Autodesk Fusion 360 part; units mm, degrees
(part 5 of 18)
  arc A132 (38.8971, -63.5184) -> (40.0971, -63.5184) centre (39.4971, -63.5184) ccw
  arc A133 (40.0971, -63.5184) -> (38.8971, -63.5184) centre (39.4971, -63.5184) ccw
  arc A134 (43.5971, -80.3272) -> (42.3971, -80.3272) centre (42.9971, -80.3272) ccw
  arc A135 (42.3971, -80.3272) -> (43.5971, -80.3272) centre (42.9971, -80.3272) ccw
  arc A136 (38.8971, -82.5812) -> (40.0971, -82.5812) centre (39.4971, -82.5812) ccw
  arc A137 (40.0971, -82.5812) -> (38.8971, -82.5812) centre (39.4971, -82.5812) ccw
  arc A138 (24.547, -80.3272) -> (23.347, -80.3272) centre (23.947, -80.3272) ccw
  arc A139 (23.347, -80.3272) -> (24.547, -80.3272) centre (23.947, -80.3272) ccw
  arc A140 (21.047, -82.5812) -> (19.847, -82.5812) centre (20.447, -82.5812) ccw
  arc A141 (19.847, -82.5812) -> (21.047, -82.5812) centre (20.447, -82.5812) ccw
  arc A142 (5.497, -80.3272) -> (4.297, -80.3272) centre (4.897, -80.3272) ccw
  arc A143 (4.297, -80.3272) -> (5.497, -80.3272) centre (4.897, -80.3272) ccw
  arc A144 (0.797, -82.5812) -> (1.997, -82.5812) centre (1.397, -82.5812) ccw
  arc A145 (1.997, -82.5812) -> (0.797, -82.5812) centre (1.397, -82.5812) ccw
  arc A146 (62.6471, -23.1516) -> (61.4471, -23.1516) centre (62.0471, -23.1516) ccw
  arc A147 (61.4471, -23.1516) -> (62.6471, -23.1516) centre (62.0471, -23.1516) ccw
  arc A148 (57.9471, -25.4057) -> (59.1471, -25.4057) centre (58.5471, -25.4057) ccw
  arc A149 (59.1471, -25.4057) -> (57.9471, -25.4057) centre (58.5471, -25.4057) ccw
  arc A150 (42.3971, -42.2017) -> (43.5971, -42.2017) centre (42.9971, -42.2017) ccw
  arc A151 (43.5971, -42.2017) -> (42.3971, -42.2017) centre (42.9971, -42.2017) ccw
  arc A152 (38.8971, -44.4557) -> (40.0971, -44.4557) centre (39.4971, -44.4557) ccw
  arc A153 (40.0971, -44.4557) -> (38.8971, -44.4557) centre (39.4971, -44.4557) ccw
  arc A154 (43.5971, -23.1516) -> (42.3971, -23.1516) centre (42.9971, -23.1516) ccw
  arc A155 (42.3971, -23.1516) -> (43.5971, -23.1516) centre (42.9971, -23.1516) ccw
  arc A156 (40.0971, -25.4057) -> (38.8971, -25.4057) centre (39.4971, -25.4057) ccw
  arc A157 (38.8971, -25.4057) -> (40.0971, -25.4057) centre (39.4971, -25.4057) ccw
  arc A158 (24.547, -23.1516) -> (23.347, -23.1516) centre (23.947, -23.1516) ccw
  arc A159 (23.347, -23.1516) -> (24.547, -23.1516) centre (23.947, -23.1516) ccw
  arc A160 (21.047, -25.4057) -> (19.847, -25.4057) centre (20.447, -25.4057) ccw
  arc A161 (19.847, -25.4057) -> (21.047, -25.4057) centre (20.447, -25.4057) ccw
  arc A162 (24.547, -61.2644) -> (23.347, -61.2644) centre (23.947, -61.2644) ccw
  arc A163 (23.347, -61.2644) -> (24.547, -61.2644) centre (23.947, -61.2644) ccw
  arc A164 (19.847, -63.5184) -> (21.047, -63.5184) centre (20.447, -63.5184) ccw
  arc A165 (21.047, -63.5184) -> (19.847, -63.5184) centre (20.447, -63.5184) ccw
  arc A166 (24.547, -42.2017) -> (23.347, -42.2017) centre (23.947, -42.2017) ccw
  arc A167 (23.347, -42.2017) -> (24.547, -42.2017) centre (23.947, -42.2017) ccw
  arc A168 (19.847, -44.4557) -> (21.047, -44.4557) centre (20.447, -44.4557) ccw
  arc A169 (21.047, -44.4557) -> (19.847, -44.4557) centre (20.447, -44.4557) ccw
  arc A170 (4.297, -23.1516) -> (5.497, -23.1516) centre (4.897, -23.1516) ccw
  arc A171 (5.497, -23.1516) -> (4.297, -23.1516) centre (4.897, -23.1516) ccw
  arc A172 (0.797, -25.4057) -> (1.997, -25.4057) centre (1.397, -25.4057) ccw
  arc A173 (1.997, -25.4057) -> (0.797, -25.4057) centre (1.397, -25.4057) ccw
  arc A174 (5.497, -42.2017) -> (4.297, -42.2017) centre (4.897, -42.2017) ccw
  arc A175 (4.297, -42.2017) -> (5.497, -42.2017) centre (4.897, -42.2017) ccw
  arc A176 (0.797, -44.4557) -> (1.997, -44.4557) centre (1.397, -44.4557) ccw
  arc A177 (1.997, -44.4557) -> (0.797, -44.4557) centre (1.397, -44.4557) ccw
  arc A178 (5.497, -61.2644) -> (4.297, -61.2644) centre (4.897, -61.2644) ccw
  arc A179 (4.297, -61.2644) -> (5.497, -61.2644) centre (4.897, -61.2644) ccw
  arc A180 (0.797, -63.5184) -> (1.997, -63.5184) centre (1.397, -63.5184) ccw
  arc A181 (1.997, -63.5184) -> (0.797, -63.5184) centre (1.397, -63.5184) ccw
  arc A182 (215.0474, -61.2644) -> (213.8474, -61.2644) centre (214.4474, -61.2644) ccw
  arc A183 (213.8474, -61.2644) -> (215.0474, -61.2644) centre (214.4474, -61.2644) ccw
  arc A184 (210.3474, -63.5184) -> (211.5474, -63.5184) centre (210.9474, -63.5184) ccw
  arc A185 (211.5474, -63.5184) -> (210.3474, -63.5184) centre (210.9474, -63.5184) ccw
  arc A186 (213.8474, -42.2017) -> (215.0474, -42.2017) centre (214.4474, -42.2017) ccw
  arc A187 (215.0474, -42.2017) -> (213.8474, -42.2017) centre (214.4474, -42.2017) ccw
  arc A188 (210.3474, -44.4557) -> (211.5474, -44.4557) centre (210.9474, -44.4557) ccw
  arc A189 (211.5474, -44.4557) -> (210.3474, -44.4557) centre (210.9474, -44.4557) ccw
  arc A190 (213.8474, -23.1516) -> (215.0474, -23.1516) centre (214.4474, -23.1516) ccw
  arc A191 (215.0474, -23.1516) -> (213.8474, -23.1516) centre (214.4474, -23.1516) ccw
  arc A192 (211.5474, -25.4057) -> (210.3474, -25.4057) centre (210.9474, -25.4057) ccw
  arc A193 (210.3474, -25.4057) -> (211.5474, -25.4057) centre (210.9474, -25.4057) ccw
  arc A194 (215.0474, -80.3272) -> (213.8474, -80.3272) centre (214.4474, -80.3272) ccw
  arc A195 (213.8474, -80.3272) -> (215.0474, -80.3272) centre (214.4474, -80.3272) ccw
  arc A196 (210.3474, -82.5812) -> (211.5474, -82.5812) centre (210.9474, -82.5812) ccw
  arc A197 (211.5474, -82.5812) -> (210.3474, -82.5812) centre (210.9474, -82.5812) ccw
  arc A198 (194.7974, -42.2017) -> (195.9974, -42.2017) centre (195.3974, -42.2017) ccw
  arc A199 (195.9974, -42.2017) -> (194.7974, -42.2017) centre (195.3974, -42.2017) ccw
  arc A200 (191.2974, -44.4557) -> (192.4974, -44.4557) centre (191.8974, -44.4557) ccw
  arc A201 (192.4974, -44.4557) -> (191.2974, -44.4557) centre (191.8974, -44.4557) ccw
  arc A202 (176.9224, -4.318) -> (175.1224, -4.318) centre (176.0224, -4.318) ccw
  arc A203 (175.1224, -4.318) -> (176.9224, -4.318) centre (176.0224, -4.318) ccw
  line L3366 (172.5823, -5.218) -> (172.5823, -3.418)
  line L3367 (174.3823, -3.418) -> (174.3823, -5.218)
  line L3368 (172.5823, -3.418) -> (174.3823, -3.418)
  line L3369 (174.3823, -5.218) -> (172.5823, -5.218)
  line L3370 (190.2943, -3.2705) -> (190.5139, -3.4901)
  line L3371 (190.2943, -5.4097) -> (189.9943, -5.4901)
  line L3372 (190.5943, -3.7901) -> (190.5943, -4.8901)
  line L3373 (189.4747, -3.4901) -> (189.6943, -3.2705)
  line L3374 (189.9943, -5.4901) -> (189.6943, -5.4097)
  line L3375 (189.3943, -3.7901) -> (189.4747, -3.4901)
  line L3376 (190.5139, -3.4901) -> (190.5943, -3.7901)
  line L3377 (189.6943, -5.4097) -> (189.4747, -5.1901)
  line L3378 (189.6943, -3.2705) -> (189.9943, -3.1901)
  line L3379 (189.9943, -3.1901) -> (190.2943, -3.2705)
  line L3380 (189.4747, -5.1901) -> (189.3943, -4.8901)
  line L3381 (189.3943, -4.8901) -> (189.3943, -3.7901)
  line L3382 (190.5139, -5.1901) -> (190.2943, -5.4097)
  line L3383 (190.5943, -4.8901) -> (190.5139, -5.1901)
  line L3384 (180.7544, -4.8901) -> (180.7544, -3.7901)
  line L3385 (181.0545, -3.2705) -> (181.3545, -3.1901)
  line L3386 (181.6545, -3.2705) -> (181.8741, -3.4901)
  line L3387 (181.8741, -5.1901) -> (181.6545, -5.4097)
  line L3388 (181.3545, -5.4901) -> (181.0545, -5.4097)
  line L3389 (180.8348, -5.1901) -> (180.7544, -4.8901)
  line L3390 (180.7544, -3.7901) -> (180.8348, -3.4901)
  line L3391 (181.3545, -3.1901) -> (181.6545, -3.2705)
  line L3392 (181.6545, -5.4097) -> (181.3545, -5.4901)
  line L3393 (181.8741, -3.4901) -> (181.9545, -3.7901)
  line L3394 (180.8348, -3.4901) -> (181.0545, -3.2705)
  line L3395 (181.0545, -5.4097) -> (180.8348, -5.1901)
  line L3396 (181.9545, -3.7901) -> (181.9545, -4.8901)
  line L3397 (181.9545, -4.8901) -> (181.8741, -5.1901)
  line L3398 (189.6943, -1.1096) -> (189.4747, -0.89)
  line L3399 (189.4747, 0.51) -> (189.6943, 0.7297)
  line L3400 (190.2943, 0.7297) -> (190.5139, 0.51)
  line L3401 (189.3943, -0.59) -> (189.3943, 0.21)
  line L3402 (189.4747, -0.89) -> (189.3943, -0.59)
  line L3403 (190.5943, -0.59) -> (190.5139, -0.89)
  line L3404 (190.2943, -1.1096) -> (189.9943, -1.19)
  line L3405 (189.3943, 0.21) -> (189.4747, 0.51)
  line L3406 (189.6943, 0.7297) -> (189.9943, 0.81)
  line L3407 (190.5139, 0.51) -> (190.5943, 0.21)
  line L3408 (189.9943, -1.19) -> (189.6943, -1.1096)
  line L3409 (190.5139, -0.89) -> (190.2943, -1.1096)
  line L3410 (190.5943, 0.21) -> (190.5943, -0.59)
  line L3411 (189.9943, 0.81) -> (190.2943, 0.7297)
  line L3412 (180.8348, -0.89) -> (180.7544, -0.59)
  line L3413 (181.0545, 0.7297) -> (181.3545, 0.81)
  line L3414 (181.9545, -0.59) -> (181.8741, -0.89)
  line L3415 (181.6545, -1.1096) -> (181.3545, -1.19)
  line L3416 (181.3545, -1.19) -> (181.0545, -1.1096)
  line L3417 (181.0545, -1.1096) -> (180.8348, -0.89)
  line L3418 (181.6545, 0.7297) -> (181.8741, 0.51)
  line L3419 (180.7544, 0.21) -> (180.8348, 0.51)
  line L3420 (181.8741, 0.51) -> (181.9545, 0.21)
  line L3421 (181.9545, 0.21) -> (181.9545, -0.59)
  line L3422 (180.8348, 0.51) -> (181.0545, 0.7297)
  line L3423 (181.8741, -0.89) -> (181.6545, -1.1096)
  line L3424 (181.3545, 0.81) -> (181.6545, 0.7297)
  line L3425 (180.7544, -0.59) -> (180.7544, 0.21)
  arc A204 (10.6139, -8.0011) -> (8.7123, -8.0011) centre (9.6631, -8.0011) ccw
  arc A205 (8.7123, -8.0011) -> (10.6139, -8.0011) centre (9.6631, -8.0011) ccw
  line L3426 (10.6139, -8.0011) -> (10.6139, -8.0011)
  line L3427 (10.6139, -5.4611) -> (10.6139, -5.4611)
  arc A206 (10.6139, -5.4611) -> (8.7123, -5.4611) centre (9.6631, -5.4611) ccw
  arc A207 (8.7123, -5.4611) -> (10.6139, -5.4611) centre (9.6631, -5.4611) ccw
  arc A208 (10.6139, -2.9211) -> (8.7123, -2.9211) centre (9.6631, -2.9211) ccw
  arc A209 (8.7123, -2.9211) -> (10.6139, -2.9211) centre (9.6631, -2.9211) ccw
  line L3428 (10.6139, -2.9211) -> (10.6139, -2.9211)
  arc A210 (-5.7879, -8.0011) -> (-3.8863, -8.0011) centre (-4.8371, -8.0011) ccw
  arc A211 (-3.8863, -8.0011) -> (-5.7879, -8.0011) centre (-4.8371, -8.0011) ccw
  arc A212 (-3.8863, -2.9211) -> (-5.7879, -2.9211) centre (-4.8371, -2.9211) ccw
  arc A213 (-5.7879, -2.9211) -> (-3.8863, -2.9211) centre (-4.8371, -2.9211) ccw
  line L3429 (4.2137, 0.039) -> (4.1223, -0.4205)
  line L3430 (4.1223, 0.4985) -> (4.2137, 0.039)
  line L3431 (3.4725, 1.1484) -> (3.862, 0.8881)
  line L3432 (0.4638, 0.8881) -> (0.8534, 1.1484)
  line L3433 (3.0129, -1.1618) -> (1.3129, -1.1618)
  line L3434 (0.8534, 1.1484) -> (1.3129, 1.2398)
  line L3435 (3.4725, -1.0704) -> (3.0129, -1.1618)
  line L3436 (0.4638, -0.8101) -> (0.2035, -0.4205)
  line L3437 (3.862, 0.8881) -> (4.1223, 0.4985)
  line L3438 (0.1121, 0.039) -> (0.2035, 0.4985)
  line L3439 (0.2035, 0.4985) -> (0.4638, 0.8881)
  line L3440 (0.8534, -1.0704) -> (0.4638, -0.8101)
  line L3441 (1.3129, 1.2398) -> (3.0129, 1.2398)
  line L3442 (4.1223, -0.4205) -> (3.862, -0.8101)
  line L3443 (1.3129, -1.1618) -> (0.8534, -1.0704)
  line L3444 (3.862, -0.8101) -> (3.4725, -1.0704)
  line L3445 (3.0129, 1.2398) -> (3.4725, 1.1484)
  line L3446 (0.2035, -0.4205) -> (0.1121, 0.039)
  line L3447 (3.4725, -9.8516) -> (3.862, -10.1119)
  line L3448 (0.1121, -10.961) -> (0.2035, -10.5015)
  line L3449 (0.8534, -9.8516) -> (1.3129, -9.7602)
  line L3450 (1.3129, -12.1618) -> (0.8534, -12.0704)
  line L3451 (0.4638, -10.1119) -> (0.8534, -9.8516)
  line L3452 (1.3129, -9.7602) -> (3.0129, -9.7602)
  line L3453 (0.8534, -12.0704) -> (0.4638, -11.8101)
  line L3454 (3.4725, -12.0704) -> (3.0129, -12.1618)
  line L3455 (3.0129, -9.7602) -> (3.4725, -9.8516)
  line L3456 (4.1223, -11.4205) -> (3.862, -11.8101)
  line L3457 (4.2137, -10.961) -> (4.1223, -11.4205)
  line L3458 (0.4638, -11.8101) -> (0.2035, -11.4205)
  line L3459 (3.0129, -12.1618) -> (1.3129, -12.1618)
  line L3460 (0.2035, -11.4205) -> (0.1121, -10.961)
  line L3461 (3.862, -10.1119) -> (4.1223, -10.5015)
  line L3462 (0.2035, -10.5015) -> (0.4638, -10.1119)
  line L3463 (4.1223, -10.5015) -> (4.2137, -10.961)
  line L3464 (3.862, -11.8101) -> (3.4725, -12.0704)
  arc A214 (196.0482, -61.2644) -> (194.7466, -61.2644) centre (195.3974, -61.2644) ccw
  arc A215 (194.7466, -61.2644) -> (196.0482, -61.2644) centre (195.3974, -61.2644) ccw
  arc A216 (191.2466, -63.5184) -> (192.5482, -63.5184) centre (191.8974, -63.5184) ccw
  arc A217 (192.5482, -63.5184) -> (191.2466, -63.5184) centre (191.8974, -63.5184) ccw
  arc A218 (175.6966, -80.3272) -> (176.9982, -80.3272) centre (176.3474, -80.3272) ccw
  arc A219 (176.9982, -80.3272) -> (175.6966, -80.3272) centre (176.3474, -80.3272) ccw
  arc A220 (172.1965, -82.5812) -> (173.4981, -82.5812) centre (172.8473, -82.5812) ccw
  arc A221 (173.4981, -82.5812) -> (172.1965, -82.5812) centre (172.8473, -82.5812) ccw
  arc A222 (175.6966, -61.2644) -> (176.9982, -61.2644) centre (176.3474, -61.2644) ccw
  arc A223 (176.9982, -61.2644) -> (175.6966, -61.2644) centre (176.3474, -61.2644) ccw
  arc A224 (173.4981, -63.5184) -> (172.1965, -63.5184) centre (172.8473, -63.5184) ccw
  arc A225 (172.1965, -63.5184) -> (173.4981, -63.5184) centre (172.8473, -63.5184) ccw
  arc A226 (176.9982, -42.2017) -> (175.6966, -42.2017) centre (176.3474, -42.2017) ccw
  arc A227 (175.6966, -42.2017) -> (176.9982, -42.2017) centre (176.3474, -42.2017) ccw
  arc A228 (172.1965, -44.4557) -> (173.4981, -44.4557) centre (172.8473, -44.4557) ccw
  arc A229 (173.4981, -44.4557) -> (172.1965, -44.4557) centre (172.8473, -44.4557) ccw
  arc A230 (176.9982, -23.1516) -> (175.6966, -23.1516) centre (176.3474, -23.1516) ccw
  arc A231 (175.6966, -23.1516) -> (176.9982, -23.1516) centre (176.3474, -23.1516) ccw
  arc A232 (172.1965, -25.4057) -> (173.4981, -25.4057) centre (172.8473, -25.4057) ccw
  arc A233 (173.4981, -25.4057) -> (172.1965, -25.4057) centre (172.8473, -25.4057) ccw
  arc A234 (157.9481, -80.3272) -> (156.6465, -80.3272) centre (157.2973, -80.3272) ccw
  arc A235 (156.6465, -80.3272) -> (157.9481, -80.3272) centre (157.2973, -80.3272) ccw
  arc A236 (153.1465, -82.5812) -> (154.4481, -82.5812) centre (153.7973, -82.5812) ccw
  arc A237 (154.4481, -82.5812) -> (153.1465, -82.5812) centre (153.7973, -82.5812) ccw
  arc A238 (157.9481, -42.2017) -> (156.6465, -42.2017) centre (157.2973, -42.2017) ccw
  arc A239 (156.6465, -42.2017) -> (157.9481, -42.2017) centre (157.2973, -42.2017) ccw
  arc A240 (154.4481, -44.4557) -> (153.1465, -44.4557) centre (153.7973, -44.4557) ccw
  arc A241 (153.1465, -44.4557) -> (154.4481, -44.4557) centre (153.7973, -44.4557) ccw
  arc A242 (157.9481, -61.2644) -> (156.6465, -61.2644) centre (157.2973, -61.2644) ccw
  arc A243 (156.6465, -61.2644) -> (157.9481, -61.2644) centre (157.2973, -61.2644) ccw
  arc A244 (154.4481, -63.5184) -> (153.1465, -63.5184) centre (153.7973, -63.5184) ccw
  arc A245 (153.1465, -63.5184) -> (154.4481, -63.5184) centre (153.7973, -63.5184) ccw
  arc A246 (156.6465, -23.1516) -> (157.9481, -23.1516) centre (157.2973, -23.1516) ccw
  arc A247 (157.9481, -23.1516) -> (156.6465, -23.1516) centre (157.2973, -23.1516) ccw
  arc A248 (154.4481, -25.4057) -> (153.1465, -25.4057) centre (153.7973, -25.4057) ccw
  arc A249 (153.1465, -25.4057) -> (154.4481, -25.4057) centre (153.7973, -25.4057) ccw
  arc A250 (138.8981, -61.2644) -> (137.5965, -61.2644) centre (138.2473, -61.2644) ccw
  arc A251 (137.5965, -61.2644) -> (138.8981, -61.2644) centre (138.2473, -61.2644) ccw
  arc A252 (134.0965, -63.5184) -> (135.3981, -63.5184) centre (134.7473, -63.5184) ccw
  arc A253 (135.3981, -63.5184) -> (134.0965, -63.5184) centre (134.7473, -63.5184) ccw
  arc A254 (138.8981, -42.2017) -> (137.5965, -42.2017) centre (138.2473, -42.2017) ccw
  arc A255 (137.5965, -42.2017) -> (138.8981, -42.2017) centre (138.2473, -42.2017) ccw
  arc A256 (134.0965, -44.4557) -> (135.3981, -44.4557) centre (134.7473, -44.4557) ccw
  arc A257 (135.3981, -44.4557) -> (134.0965, -44.4557) centre (134.7473, -44.4557) ccw
  arc A258 (138.8981, -23.1516) -> (137.5965, -23.1516) centre (138.2473, -23.1516) ccw
  arc A259 (137.5965, -23.1516) -> (138.8981, -23.1516) centre (138.2473, -23.1516) ccw
  arc A260 (134.0965, -25.4057) -> (135.3981, -25.4057) centre (134.7473, -25.4057) ccw
  arc A261 (135.3981, -25.4057) -> (134.0965, -25.4057) centre (134.7473, -25.4057) ccw
  arc A262 (138.8981, -80.3272) -> (137.5965, -80.3272) centre (138.2473, -80.3272) ccw
  arc A263 (137.5965, -80.3272) -> (138.8981, -80.3272) centre (138.2473, -80.3272) ccw
  arc A264 (135.3981, -82.5812) -> (134.0965, -82.5812) centre (134.7473, -82.5812) ccw
  arc A265 (134.0965, -82.5812) -> (135.3981, -82.5812) centre (134.7473, -82.5812) ccw
  arc A266 (119.848, -80.3272) -> (118.5464, -80.3272) centre (119.1972, -80.3272) ccw
  arc A267 (118.5464, -80.3272) -> (119.848, -80.3272) centre (119.1972, -80.3272) ccw
  arc A268 (115.0464, -82.5812) -> (116.348, -82.5812) centre (115.6972, -82.5812) ccw
  arc A269 (116.348, -82.5812) -> (115.0464, -82.5812) centre (115.6972, -82.5812) ccw
  arc A270 (118.5464, -61.2644) -> (119.848, -61.2644) centre (119.1972, -61.2644) ccw
  arc A271 (119.848, -61.2644) -> (118.5464, -61.2644) centre (119.1972, -61.2644) ccw
  arc A272 (115.0464, -63.5184) -> (116.348, -63.5184) centre (115.6972, -63.5184) ccw
  arc A273 (116.348, -63.5184) -> (115.0464, -63.5184) centre (115.6972, -63.5184) ccw
  arc A274 (118.5464, -23.1516) -> (119.848, -23.1516) centre (119.1972, -23.1516) ccw
  arc A275 (119.848, -23.1516) -> (118.5464, -23.1516) centre (119.1972, -23.1516) ccw
  arc A276 (115.0464, -25.4057) -> (116.348, -25.4057) centre (115.6972, -25.4057) ccw
  arc A277 (116.348, -25.4057) -> (115.0464, -25.4057) centre (115.6972, -25.4057) ccw
  arc A278 (118.5464, -42.2017) -> (119.848, -42.2017) centre (119.1972, -42.2017) ccw
  arc A279 (119.848, -42.2017) -> (118.5464, -42.2017) centre (119.1972, -42.2017) ccw
  arc A280 (115.0464, -44.4557) -> (116.348, -44.4557) centre (115.6972, -44.4557) ccw
  arc A281 (116.348, -44.4557) -> (115.0464, -44.4557) centre (115.6972, -44.4557) ccw
  arc A282 (99.4964, -23.1516) -> (100.798, -23.1516) centre (100.1472, -23.1516) ccw
  arc A283 (100.798, -23.1516) -> (99.4964, -23.1516) centre (100.1472, -23.1516) ccw
  arc A284 (97.298, -25.4057) -> (95.9964, -25.4057) centre (96.6472, -25.4057) ccw
  arc A285 (95.9964, -25.4057) -> (97.298, -25.4057) centre (96.6472, -25.4057) ccw
  arc A286 (100.798, -42.2017) -> (99.4964, -42.2017) centre (100.1472, -42.2017) ccw
  arc A287 (99.4964, -42.2017) -> (100.798, -42.2017) centre (100.1472, -42.2017) ccw
  arc A288 (97.298, -44.4557) -> (95.9964, -44.4557) centre (96.6472, -44.4557) ccw
  arc A289 (95.9964, -44.4557) -> (97.298, -44.4557) centre (96.6472, -44.4557) ccw
  arc A290 (99.4964, -80.3272) -> (100.798, -80.3272) centre (100.1472, -80.3272) ccw
  arc A291 (100.798, -80.3272) -> (99.4964, -80.3272) centre (100.1472, -80.3272) ccw
  arc A292 (95.9964, -82.5812) -> (97.298, -82.5812) centre (96.6472, -82.5812) ccw
  arc A293 (97.298, -82.5812) -> (95.9964, -82.5812) centre (96.6472, -82.5812) ccw
  arc A294 (99.4964, -61.2644) -> (100.798, -61.2644) centre (100.1472, -61.2644) ccw
  arc A295 (100.798, -61.2644) -> (99.4964, -61.2644) centre (100.1472, -61.2644) ccw
  arc A296 (95.9964, -63.5184) -> (97.298, -63.5184) centre (96.6472, -63.5184) ccw
  arc A297 (97.298, -63.5184) -> (95.9964, -63.5184) centre (96.6472, -63.5184) ccw
  arc A298 (196.0482, -80.3272) -> (194.7466, -80.3272) centre (195.3974, -80.3272) ccw
  arc A299 (194.7466, -80.3272) -> (196.0482, -80.3272) centre (195.3974, -80.3272) ccw
  arc A300 (191.2466, -82.5812) -> (192.5482, -82.5812) centre (191.8974, -82.5812) ccw
  arc A301 (192.5482, -82.5812) -> (191.2466, -82.5812) centre (191.8974, -82.5812) ccw
  arc A302 (196.0482, -23.1516) -> (194.7466, -23.1516) centre (195.3974, -23.1516) ccw
  arc A303 (194.7466, -23.1516) -> (196.0482, -23.1516) centre (195.3974, -23.1516) ccw
  arc A304 (191.2466, -25.4057) -> (192.5482, -25.4057) centre (191.8974, -25.4057) ccw
  arc A305 (192.5482, -25.4057) -> (191.2466, -25.4057) centre (191.8974, -25.4057) ccw
  arc A306 (80.4464, -80.3272) -> (81.748, -80.3272) centre (81.0972, -80.3272) ccw
  arc A307 (81.748, -80.3272) -> (80.4464, -80.3272) centre (81.0972, -80.3272) ccw
  arc A308 (76.9464, -82.5812) -> (78.248, -82.5812) centre (77.5972, -82.5812) ccw
  arc A309 (78.248, -82.5812) -> (76.9464, -82.5812) centre (77.5972, -82.5812) ccw
  arc A310 (80.4464, -42.2017) -> (81.748, -42.2017) centre (81.0972, -42.2017) ccw
  arc A311 (81.748, -42.2017) -> (80.4464, -42.2017) centre (81.0972, -42.2017) ccw
  arc A312 (78.248, -44.4557) -> (76.9464, -44.4557) centre (77.5972, -44.4557) ccw
  arc A313 (76.9464, -44.4557) -> (78.248, -44.4557) centre (77.5972, -44.4557) ccw
  arc A314 (80.4464, -23.1516) -> (81.748, -23.1516) centre (81.0972, -23.1516) ccw
  arc A315 (81.748, -23.1516) -> (80.4464, -23.1516) centre (81.0972, -23.1516) ccw
  arc A316 (78.248, -25.4057) -> (76.9464, -25.4057) centre (77.5972, -25.4057) ccw
  arc A317 (76.9464, -25.4057) -> (78.248, -25.4057) centre (77.5972, -25.4057) ccw
  arc A318 (80.4464, -61.2644) -> (81.748, -61.2644) centre (81.0972, -61.2644) ccw
  arc A319 (81.748, -61.2644) -> (80.4464, -61.2644) centre (81.0972, -61.2644) ccw
  arc A320 (76.9464, -63.5184) -> (78.248, -63.5184) centre (77.5972, -63.5184) ccw
  arc A321 (78.248, -63.5184) -> (76.9464, -63.5184) centre (77.5972, -63.5184) ccw
  arc A322 (61.3963, -80.3272) -> (62.6979, -80.3272) centre (62.0471, -80.3272) ccw
  arc A323 (62.6979, -80.3272) -> (61.3963, -80.3272) centre (62.0471, -80.3272) ccw
  arc A324 (57.8963, -82.5812) -> (59.1979, -82.5812) centre (58.5471, -82.5812) ccw
  arc A325 (59.1979, -82.5812) -> (57.8963, -82.5812) centre (58.5471, -82.5812) ccw
  arc A326 (62.6979, -61.2644) -> (61.3963, -61.2644) centre (62.0471, -61.2644) ccw
  arc A327 (61.3963, -61.2644) -> (62.6979, -61.2644) centre (62.0471, -61.2644) ccw
  arc A328 (59.1979, -63.5184) -> (57.8963, -63.5184) centre (58.5471, -63.5184) ccw
  arc A329 (57.8963, -63.5184) -> (59.1979, -63.5184) centre (58.5471, -63.5184) ccw
  arc A330 (61.3963, -42.2017) -> (62.6979, -42.2017) centre (62.0471, -42.2017) ccw
  arc A331 (62.6979, -42.2017) -> (61.3963, -42.2017) centre (62.0471, -42.2017) ccw
  arc A332 (57.8963, -44.4557) -> (59.1979, -44.4557) centre (58.5471, -44.4557) ccw
  arc A333 (59.1979, -44.4557) -> (57.8963, -44.4557) centre (58.5471, -44.4557) ccw
  arc A334 (42.3463, -61.2644) -> (43.6479, -61.2644) centre (42.9971, -61.2644) ccw
  arc A335 (43.6479, -61.2644) -> (42.3463, -61.2644) centre (42.9971, -61.2644) ccw
  arc A336 (40.1479, -63.5184) -> (38.8463, -63.5184) centre (39.4971, -63.5184) ccw
  arc A337 (38.8463, -63.5184) -> (40.1479, -63.5184) centre (39.4971, -63.5184) ccw
  arc A338 (42.3463, -80.3272) -> (43.6479, -80.3272) centre (42.9971, -80.3272) ccw
  arc A339 (43.6479, -80.3272) -> (42.3463, -80.3272) centre (42.9971, -80.3272) ccw
  arc A340 (38.8463, -82.5812) -> (40.1479, -82.5812) centre (39.4971, -82.5812) ccw
  arc A341 (40.1479, -82.5812) -> (38.8463, -82.5812) centre (39.4971, -82.5812) ccw
  arc A342 (23.2962, -80.3272) -> (24.5978, -80.3272) centre (23.947, -80.3272) ccw
  arc A343 (24.5978, -80.3272) -> (23.2962, -80.3272) centre (23.947, -80.3272) ccw
  arc A344 (19.7962, -82.5812) -> (21.0978, -82.5812) centre (20.447, -82.5812) ccw
  arc A345 (21.0978, -82.5812) -> (19.7962, -82.5812) centre (20.447, -82.5812) ccw
  arc A346 (5.5478, -80.3272) -> (4.2462, -80.3272) centre (4.897, -80.3272) ccw
  arc A347 (4.2462, -80.3272) -> (5.5478, -80.3272) centre (4.897, -80.3272) ccw
  arc A348 (0.7462, -82.5812) -> (2.0478, -82.5812) centre (1.397, -82.5812) ccw
  arc A349 (2.0478, -82.5812) -> (0.7462, -82.5812) centre (1.397, -82.5812) ccw
  arc A350 (61.3963, -23.1516) -> (62.6979, -23.1516) centre (62.0471, -23.1516) ccw
  arc A351 (62.6979, -23.1516) -> (61.3963, -23.1516) centre (62.0471, -23.1516) ccw
  arc A352 (59.1979, -25.4057) -> (57.8963, -25.4057) centre (58.5471, -25.4057) ccw
  arc A353 (57.8963, -25.4057) -> (59.1979, -25.4057) centre (58.5471, -25.4057) ccw
  arc A354 (43.6479, -42.2017) -> (42.3463, -42.2017) centre (42.9971, -42.2017) ccw
  arc A355 (42.3463, -42.2017) -> (43.6479, -42.2017) centre (42.9971, -42.2017) ccw
  arc A356 (38.8463, -44.4557) -> (40.1479, -44.4557) centre (39.4971, -44.4557) ccw
  arc A357 (40.1479, -44.4557) -> (38.8463, -44.4557) centre (39.4971, -44.4557) ccw
  arc A358 (43.6479, -23.1516) -> (42.3463, -23.1516) centre (42.9971, -23.1516) ccw
  arc A359 (42.3463, -23.1516) -> (43.6479, -23.1516) centre (42.9971, -23.1516) ccw
  arc A360 (38.8463, -25.4057) -> (40.1479, -25.4057) centre (39.4971, -25.4057) ccw
  arc A361 (40.1479, -25.4057) -> (38.8463, -25.4057) centre (39.4971, -25.4057) ccw
  arc A362 (23.2962, -23.1516) -> (24.5978, -23.1516) centre (23.947, -23.1516) ccw
  arc A363 (24.5978, -23.1516) -> (23.2962, -23.1516) centre (23.947, -23.1516) ccw
  arc A364 (21.0978, -25.4057) -> (19.7962, -25.4057) centre (20.447, -25.4057) ccw
  arc A365 (19.7962, -25.4057) -> (21.0978, -25.4057) centre (20.447, -25.4057) ccw
  arc A366 (23.2962, -61.2644) -> (24.5978, -61.2644) centre (23.947, -61.2644) ccw
  arc A367 (24.5978, -61.2644) -> (23.2962, -61.2644) centre (23.947, -61.2644) ccw
  arc A368 (21.0978, -63.5184) -> (19.7962, -63.5184) centre (20.447, -63.5184) ccw
  arc A369 (19.7962, -63.5184) -> (21.0978, -63.5184) centre (20.447, -63.5184) ccw
  arc A370 (24.5978, -42.2017) -> (23.2962, -42.2017) centre (23.947, -42.2017) ccw
  arc A371 (23.2962, -42.2017) -> (24.5978, -42.2017) centre (23.947, -42.2017) ccw
  arc A372 (19.7962, -44.4557) -> (21.0978, -44.4557) centre (20.447, -44.4557) ccw
  arc A373 (21.0978, -44.4557) -> (19.7962, -44.4557) centre (20.447, -44.4557) ccw
  arc A374 (5.5478, -23.1516) -> (4.2462, -23.1516) centre (4.897, -23.1516) ccw
  arc A375 (4.2462, -23.1516) -> (5.5478, -23.1516) centre (4.897, -23.1516) ccw
  arc A376 (2.0478, -25.4057) -> (0.7462, -25.4057) centre (1.397, -25.4057) ccw
  arc A377 (0.7462, -25.4057) -> (2.0478, -25.4057) centre (1.397, -25.4057) ccw
  arc A378 (4.2462, -42.2017) -> (5.5478, -42.2017) centre (4.897, -42.2017) ccw
  arc A379 (5.5478, -42.2017) -> (4.2462, -42.2017) centre (4.897, -42.2017) ccw
  arc A380 (2.0478, -44.4557) -> (0.7462, -44.4557) centre (1.397, -44.4557) ccw
  arc A381 (0.7462, -44.4557) -> (2.0478, -44.4557) centre (1.397, -44.4557) ccw
  arc A382 (4.2462, -61.2644) -> (5.5478, -61.2644) centre (4.897, -61.2644) ccw
  arc A383 (5.5478, -61.2644) -> (4.2462, -61.2644) centre (4.897, -61.2644) ccw
  arc A384 (2.0478, -63.5184) -> (0.7462, -63.5184) centre (1.397, -63.5184) ccw
  arc A385 (0.7462, -63.5184) -> (2.0478, -63.5184) centre (1.397, -63.5184) ccw
  arc A386 (213.7966, -61.2644) -> (215.0982, -61.2644) centre (214.4474, -61.2644) ccw
  arc A387 (215.0982, -61.2644) -> (213.7966, -61.2644) centre (214.4474, -61.2644) ccw
  arc A388 (210.2966, -63.5184) -> (211.5982, -63.5184) centre (210.9474, -63.5184) ccw
  arc A389 (211.5982, -63.5184) -> (210.2966, -63.5184) centre (210.9474, -63.5184) ccw
  arc A390 (215.0982, -42.2017) -> (213.7966, -42.2017) centre (214.4474, -42.2017) ccw
  arc A391 (213.7966, -42.2017) -> (215.0982, -42.2017) centre (214.4474, -42.2017) ccw
  arc A392 (211.5982, -44.4557) -> (210.2966, -44.4557) centre (210.9474, -44.4557) ccw
  arc A393 (210.2966, -44.4557) -> (211.5982, -44.4557) centre (210.9474, -44.4557) ccw
  arc A394 (215.0982, -23.1516) -> (213.7966, -23.1516) centre (214.4474, -23.1516) ccw
  arc A395 (213.7966, -23.1516) -> (215.0982, -23.1516) centre (214.4474, -23.1516) ccw
  arc A396 (211.5982, -25.4057) -> (210.2966, -25.4057) centre (210.9474, -25.4057) ccw
  arc A397 (210.2966, -25.4057) -> (211.5982, -25.4057) centre (210.9474, -25.4057) ccw
  arc A398 (215.0982, -80.3272) -> (213.7966, -80.3272) centre (214.4474, -80.3272) ccw
  arc A399 (213.7966, -80.3272) -> (215.0982, -80.3272) centre (214.4474, -80.3272) ccw
  arc A400 (211.5982, -82.5812) -> (210.2966, -82.5812) centre (210.9474, -82.5812) ccw
  arc A401 (210.2966, -82.5812) -> (211.5982, -82.5812) centre (210.9474, -82.5812) ccw
  arc A402 (194.7466, -42.2017) -> (196.0482, -42.2017) centre (195.3974, -42.2017) ccw
  arc A403 (196.0482, -42.2017) -> (194.7466, -42.2017) centre (195.3974, -42.2017) ccw
  arc A404 (191.2466, -44.4557) -> (192.5482, -44.4557) centre (191.8974, -44.4557) ccw
  arc A405 (192.5482, -44.4557) -> (191.2466, -44.4557) centre (191.8974, -44.4557) ccw
  arc A406 (176.9732, -4.318) -> (175.0716, -4.318) centre (176.0224, -4.318) ccw
  arc A407 (175.0716, -4.318) -> (176.9732, -4.318) centre (176.0224, -4.318) ccw
  line L3465 (174.4331, -5.2688) -> (172.5315, -5.2688)
  line L3466 (172.5315, -5.2688) -> (172.5315, -3.3672)
  line L3467 (172.5315, -3.3672) -> (174.4331, -3.3672)
  line L3468 (174.4331, -3.3672) -> (174.4331, -5.2688)
  line L3469 (190.2693, -3.3138) -> (190.4706, -3.5151)
  line L3470 (189.4443, -3.7901) -> (189.518, -3.5151)
  line L3471 (189.9943, -3.2401) -> (190.2693, -3.3138)
  line L3472 (189.9943, -5.4401) -> (189.7193, -5.3664)
  line L3473 (189.4443, -4.8901) -> (189.4443, -3.7901)
  line L3474 (190.5443, -3.7901) -> (190.5443, -4.8901)
  line L3475 (189.518, -3.5151) -> (189.7193, -3.3138)
  line L3476 (190.5443, -4.8901) -> (190.4706, -5.1651)
  line L3477 (190.4706, -5.1651) -> (190.2693, -5.3664)
  line L3478 (190.4706, -3.5151) -> (190.5443, -3.7901)
  line L3479 (189.7193, -5.3664) -> (189.518, -5.1651)
  line L3480 (189.518, -5.1651) -> (189.4443, -4.8901)
  line L3481 (189.7193, -3.3138) -> (189.9943, -3.2401)
  line L3482 (190.2693, -5.3664) -> (189.9943, -5.4401)
  line L3483 (180.8781, -3.5151) -> (181.0795, -3.3138)
  line L3484 (181.3545, -3.2401) -> (181.6295, -3.3138)
  line L3485 (181.0795, -3.3138) -> (181.3545, -3.2401)
  line L3486 (180.8045, -3.7901) -> (180.8781, -3.5151)
  line L3487 (181.9045, -4.8901) -> (181.8308, -5.1651)
  line L3488 (181.9045, -3.7901) -> (181.9045, -4.8901)
  line L3489 (181.6295, -5.3664) -> (181.3545, -5.4401)
  line L3490 (181.0795, -5.3664) -> (180.8781, -5.1651)
  line L3491 (180.8045, -4.8901) -> (180.8045, -3.7901)
  line L3492 (181.3545, -5.4401) -> (181.0795, -5.3664)
  line L3493 (181.8308, -3.5151) -> (181.9045, -3.7901)
  line L3494 (180.8781, -5.1651) -> (180.8045, -4.8901)
  line L3495 (181.8308, -5.1651) -> (181.6295, -5.3664)
  line L3496 (181.6295, -3.3138) -> (181.8308, -3.5151)
  line L3497 (189.7193, -1.0663) -> (189.518, -0.865)
  line L3498 (189.518, 0.485) -> (189.7193, 0.6863)
  line L3499 (190.4706, 0.485) -> (190.5443, 0.21)
  line L3500 (190.2693, 0.6863) -> (190.4706, 0.485)
  line L3501 (189.518, -0.865) -> (189.4443, -0.59)
  line L3502 (189.9943, -1.14) -> (189.7193, -1.0663)
  line L3503 (190.4706, -0.865) -> (190.2693, -1.0663)
  line L3504 (190.5443, 0.21) -> (190.5443, -0.59)
  line L3505 (189.7193, 0.6863) -> (189.9943, 0.76)
  line L3506 (190.5443, -0.59) -> (190.4706, -0.865)
  line L3507 (190.2693, -1.0663) -> (189.9943, -1.14)
  line L3508 (189.4443, 0.21) -> (189.518, 0.485)
  line L3509 (189.4443, -0.59) -> (189.4443, 0.21)
  line L3510 (189.9943, 0.76) -> (190.2693, 0.6863)
  line L3511 (180.8781, 0.485) -> (181.0795, 0.6863)
  line L3512 (181.6295, -1.0663) -> (181.3545, -1.14)
  line L3513 (180.8045, -0.59) -> (180.8045, 0.21)
  line L3514 (181.9045, -0.59) -> (181.8308, -0.865)
  line L3515 (181.8308, -0.865) -> (181.6295, -1.0663)
  line L3516 (181.9045, 0.21) -> (181.9045, -0.59)
  line L3517 (181.3545, -1.14) -> (181.0795, -1.0663)
  line L3518 (180.8781, -0.865) -> (180.8045, -0.59)
  line L3519 (180.8045, 0.21) -> (180.8781, 0.485)
  line L3520 (181.6295, 0.6863) -> (181.8308, 0.485)
  line L3521 (181.3545, 0.76) -> (181.6295, 0.6863)
  line L3522 (181.0795, -1.0663) -> (180.8781, -0.865)
  line L3523 (181.8308, 0.485) -> (181.9045, 0.21)
  line L3524 (181.0795, 0.6863) -> (181.3545, 0.76)
  arc A408 (8.7631, -8.0011) -> (10.5631, -8.0011) centre (9.6631, -8.0011) ccw
  arc A409 (10.5631, -8.0011) -> (8.7631, -8.0011) centre (9.6631, -8.0011) ccw
  arc A410 (8.7631, -5.4611) -> (10.5631, -5.4611) centre (9.6631, -5.4611) ccw
  arc A411 (10.5631, -5.4611) -> (8.7631, -5.4611) centre (9.6631, -5.4611) ccw
  arc A412 (8.7631, -2.9211) -> (10.5631, -2.9211) centre (9.6631, -2.9211) ccw
  arc A413 (10.5631, -2.9211) -> (8.7631, -2.9211) centre (9.6631, -2.9211) ccw
  arc A414 (-3.9371, -8.0011) -> (-5.7371, -8.0011) centre (-4.8371, -8.0011) ccw
  line L3525 (-3.9371, -8.0011) -> (-3.9371, -8.0011)
  arc A415 (-5.7371, -8.0011) -> (-3.9371, -8.0011) centre (-4.8371, -8.0011) ccw
  arc A416 (-3.9371, -2.9211) -> (-5.7371, -2.9211) centre (-4.8371, -2.9211) ccw
  line L3526 (-3.9371, -2.9211) -> (-3.9371, -2.9211)
  arc A417 (-5.7371, -2.9211) -> (-3.9371, -2.9211) centre (-4.8371, -2.9211) ccw
  line L3527 (3.0129, -1.111) -> (1.3129, -1.111)
  line L3528 (0.8729, 1.1015) -> (1.3129, 1.189)
  line L3529 (0.1629, 0.039) -> (0.2505, 0.4791)
  line L3530 (3.0129, 1.189) -> (3.453, 1.1015)
  line L3531 (0.4998, -0.7742) -> (0.2505, -0.4011)
  line L3532 (4.0754, -0.4011) -> (3.8261, -0.7742)
  line L3533 (3.453, -1.0235) -> (3.0129, -1.111)
  line L3534 (4.1629, 0.039) -> (4.0754, -0.4011)
  line L3535 (3.8261, 0.8522) -> (4.0754, 0.4791)
  line L3536 (3.8261, -0.7742) -> (3.453, -1.0235)
  line L3537 (1.3129, -1.111) -> (0.8729, -1.0235)
  line L3538 (3.453, 1.1015) -> (3.8261, 0.8522)
  line L3539 (0.2505, 0.4791) -> (0.4998, 0.8522)
  line L3540 (1.3129, 1.189) -> (3.0129, 1.189)
  line L3541 (0.2505, -0.4011) -> (0.1629, 0.039)
  line L3542 (0.8729, -1.0235) -> (0.4998, -0.7742)
  line L3543 (0.4998, 0.8522) -> (0.8729, 1.1015)
  line L3544 (4.0754, 0.4791) -> (4.1629, 0.039)
  line L3545 (0.2505, -11.4011) -> (0.1629, -10.961)
  line L3546 (4.1629, -10.961) -> (4.0754, -11.4011)
  line L3547 (0.8729, -12.0235) -> (0.4998, -11.7742)
  line L3548 (3.8261, -10.1478) -> (4.0754, -10.5209)
  line L3549 (0.4998, -11.7742) -> (0.2505, -11.4011)
  line L3550 (4.0754, -11.4011) -> (3.8261, -11.7742)
  line L3551 (3.453, -9.8985) -> (3.8261, -10.1478)
  line L3552 (1.3129, -9.811) -> (3.0129, -9.811)
  line L3553 (3.8261, -11.7742) -> (3.453, -12.0235)
  line L3554 (0.8729, -9.8985) -> (1.3129, -9.811)
  line L3555 (0.1629, -10.961) -> (0.2505, -10.5209)
  line L3556 (3.0129, -12.111) -> (1.3129, -12.111)
  line L3557 (4.0754, -10.5209) -> (4.1629, -10.961)
  line L3558 (1.3129, -12.111) -> (0.8729, -12.0235)
  line L3559 (0.4998, -10.1478) -> (0.8729, -9.8985)
  line L3560 (3.0129, -9.811) -> (3.453, -9.8985)
  line L3561 (0.2505, -10.5209) -> (0.4998, -10.1478)
  line L3562 (3.453, -12.0235) -> (3.0129, -12.111)
  arc A418 (194.7974, -61.2644) -> (195.9974, -61.2644) centre (195.3974, -61.2644) ccw
  arc A419 (195.9974, -61.2644) -> (194.7974, -61.2644) centre (195.3974, -61.2644) ccw
  arc A420 (191.2974, -63.5184) -> (192.4974, -63.5184) centre (191.8974, -63.5184) ccw
  arc A421 (192.4974, -63.5184) -> (191.2974, -63.5184) centre (191.8974, -63.5184) ccw
  arc A422 (175.7474, -80.3272) -> (176.9474, -80.3272) centre (176.3474, -80.3272) ccw
  arc A423 (176.9474, -80.3272) -> (175.7474, -80.3272) centre (176.3474, -80.3272) ccw
  arc A424 (172.2473, -82.5812) -> (173.4473, -82.5812) centre (172.8473, -82.5812) ccw
  arc A425 (173.4473, -82.5812) -> (172.2473, -82.5812) centre (172.8473, -82.5812) ccw
  arc A426 (175.7474, -61.2644) -> (176.9474, -61.2644) centre (176.3474, -61.2644) ccw
  arc A427 (176.9474, -61.2644) -> (175.7474, -61.2644) centre (176.3474, -61.2644) ccw
  arc A428 (172.2473, -63.5184) -> (173.4473, -63.5184) centre (172.8473, -63.5184) ccw
  arc A429 (173.4473, -63.5184) -> (172.2473, -63.5184) centre (172.8473, -63.5184) ccw
  arc A430 (175.7474, -42.2017) -> (176.9474, -42.2017) centre (176.3474, -42.2017) ccw
  arc A431 (176.9474, -42.2017) -> (175.7474, -42.2017) centre (176.3474, -42.2017) ccw
  arc A432 (172.2473, -44.4557) -> (173.4473, -44.4557) centre (172.8473, -44.4557) ccw
  arc A433 (173.4473, -44.4557) -> (172.2473, -44.4557) centre (172.8473, -44.4557) ccw
  arc A434 (176.9474, -23.1516) -> (175.7474, -23.1516) centre (176.3474, -23.1516) ccw
  arc A435 (175.7474, -23.1516) -> (176.9474, -23.1516) centre (176.3474, -23.1516) ccw
  arc A436 (173.4473, -25.4057) -> (172.2473, -25.4057) centre (172.8473, -25.4057) ccw
  arc A437 (172.2473, -25.4057) -> (173.4473, -25.4057) centre (172.8473, -25.4057) ccw
  arc A438 (156.6973, -80.3272) -> (157.8973, -80.3272) centre (157.2973, -80.3272) ccw
  arc A439 (157.8973, -80.3272) -> (156.6973, -80.3272) centre (157.2973, -80.3272) ccw
  arc A440 (154.3973, -82.5812) -> (153.1973, -82.5812) centre (153.7973, -82.5812) ccw
  arc A441 (153.1973, -82.5812) -> (154.3973, -82.5812) centre (153.7973, -82.5812) ccw
  arc A442 (156.6973, -42.2017) -> (157.8973, -42.2017) centre (157.2973, -42.2017) ccw
  arc A443 (157.8973, -42.2017) -> (156.6973, -42.2017) centre (157.2973, -42.2017) ccw
  arc A444 (154.3973, -44.4557) -> (153.1973, -44.4557) centre (153.7973, -44.4557) ccw
  arc A445 (153.1973, -44.4557) -> (154.3973, -44.4557) centre (153.7973, -44.4557) ccw
  arc A446 (157.8973, -61.2644) -> (156.6973, -61.2644) centre (157.2973, -61.2644) ccw
  arc A447 (156.6973, -61.2644) -> (157.8973, -61.2644) centre (157.2973, -61.2644) ccw
  arc A448 (153.1973, -63.5184) -> (154.3973, -63.5184) centre (153.7973, -63.5184) ccw
  arc A449 (154.3973, -63.5184) -> (153.1973, -63.5184) centre (153.7973, -63.5184) ccw
  arc A450 (157.8973, -23.1516) -> (156.6973, -23.1516) centre (157.2973, -23.1516) ccw
  arc A451 (156.6973, -23.1516) -> (157.8973, -23.1516) centre (157.2973, -23.1516) ccw
  arc A452 (153.1973, -25.4057) -> (154.3973, -25.4057) centre (153.7973, -25.4057) ccw
  arc A453 (154.3973, -25.4057) -> (153.1973, -25.4057) centre (153.7973, -25.4057) ccw
  arc A454 (137.6473, -61.2644) -> (138.8473, -61.2644) centre (138.2473, -61.2644) ccw
  arc A455 (138.8473, -61.2644) -> (137.6473, -61.2644) centre (138.2473, -61.2644) ccw
  arc A456 (134.1473, -63.5184) -> (135.3473, -63.5184) centre (134.7473, -63.5184) ccw
  arc A457 (135.3473, -63.5184) -> (134.1473, -63.5184) centre (134.7473, -63.5184) ccw
  arc A458 (137.6473, -42.2017) -> (138.8473, -42.2017) centre (138.2473, -42.2017) ccw
  arc A459 (138.8473, -42.2017) -> (137.6473, -42.2017) centre (138.2473, -42.2017) ccw
  arc A460 (135.3473, -44.4557) -> (134.1473, -44.4557) centre (134.7473, -44.4557) ccw
  arc A461 (134.1473, -44.4557) -> (135.3473, -44.4557) centre (134.7473, -44.4557) ccw
  arc A462 (138.8473, -23.1516) -> (137.6473, -23.1516) centre (138.2473, -23.1516) ccw
  arc A463 (137.6473, -23.1516) -> (138.8473, -23.1516) centre (138.2473, -23.1516) ccw
  arc A464 (134.1473, -25.4057) -> (135.3473, -25.4057) centre (134.7473, -25.4057) ccw
  arc A465 (135.3473, -25.4057) -> (134.1473, -25.4057) centre (134.7473, -25.4057) ccw
  arc A466 (137.6473, -80.3272) -> (138.8473, -80.3272) centre (138.2473, -80.3272) ccw
  arc A467 (138.8473, -80.3272) -> (137.6473, -80.3272) centre (138.2473, -80.3272) ccw
  arc A468 (135.3473, -82.5812) -> (134.1473, -82.5812) centre (134.7473, -82.5812) ccw
  arc A469 (134.1473, -82.5812) -> (135.3473, -82.5812) centre (134.7473, -82.5812) ccw
  arc A470 (118.5972, -80.3272) -> (119.7972, -80.3272) centre (119.1972, -80.3272) ccw
  arc A471 (119.7972, -80.3272) -> (118.5972, -80.3272) centre (119.1972, -80.3272) ccw
  arc A472 (115.0972, -82.5812) -> (116.2972, -82.5812) centre (115.6972, -82.5812) ccw
  arc A473 (116.2972, -82.5812) -> (115.0972, -82.5812) centre (115.6972, -82.5812) ccw
  arc A474 (119.7972, -61.2644) -> (118.5972, -61.2644) centre (119.1972, -61.2644) ccw
  arc A475 (118.5972, -61.2644) -> (119.7972, -61.2644) centre (119.1972, -61.2644) ccw
  arc A476 (116.2972, -63.5184) -> (115.0972, -63.5184) centre (115.6972, -63.5184) ccw
  arc A477 (115.0972, -63.5184) -> (116.2972, -63.5184) centre (115.6972, -63.5184) ccw
  arc A478 (119.7972, -23.1516) -> (118.5972, -23.1516) centre (119.1972, -23.1516) ccw
  arc A479 (118.5972, -23.1516) -> (119.7972, -23.1516) centre (119.1972, -23.1516) ccw
  arc A480 (115.0972, -25.4057) -> (116.2972, -25.4057) centre (115.6972, -25.4057) ccw
  arc A481 (116.2972, -25.4057) -> (115.0972, -25.4057) centre (115.6972, -25.4057) ccw
  arc A482 (118.5972, -42.2017) -> (119.7972, -42.2017) centre (119.1972, -42.2017) ccw
  arc A483 (119.7972, -42.2017) -> (118.5972, -42.2017) centre (119.1972, -42.2017) ccw
  arc A484 (115.0972, -44.4557) -> (116.2972, -44.4557) centre (115.6972, -44.4557) ccw
  arc A485 (116.2972, -44.4557) -> (115.0972, -44.4557) centre (115.6972, -44.4557) ccw
  arc A486 (100.7472, -23.1516) -> (99.5472, -23.1516) centre (100.1472, -23.1516) ccw
  arc A487 (99.5472, -23.1516) -> (100.7472, -23.1516) centre (100.1472, -23.1516) ccw
  arc A488 (96.0472, -25.4057) -> (97.2472, -25.4057) centre (96.6472, -25.4057) ccw
  arc A489 (97.2472, -25.4057) -> (96.0472, -25.4057) centre (96.6472, -25.4057) ccw
  arc A490 (99.5472, -42.2017) -> (100.7472, -42.2017) centre (100.1472, -42.2017) ccw
  arc A491 (100.7472, -42.2017) -> (99.5472, -42.2017) centre (100.1472, -42.2017) ccw
  arc A492 (96.0472, -44.4557) -> (97.2472, -44.4557) centre (96.6472, -44.4557) ccw
  arc A493 (97.2472, -44.4557) -> (96.0472, -44.4557) centre (96.6472, -44.4557) ccw
  arc A494 (100.7472, -80.3272) -> (99.5472, -80.3272) centre (100.1472, -80.3272) ccw
  arc A495 (99.5472, -80.3272) -> (100.7472, -80.3272) centre (100.1472, -80.3272) ccw
  arc A496 (96.0472, -82.5812) -> (97.2472, -82.5812) centre (96.6472, -82.5812) ccw
  arc A497 (97.2472, -82.5812) -> (96.0472, -82.5812) centre (96.6472, -82.5812) ccw
  arc A498 (99.5472, -61.2644) -> (100.7472, -61.2644) centre (100.1472, -61.2644) ccw
  arc A499 (100.7472, -61.2644) -> (99.5472, -61.2644) centre (100.1472, -61.2644) ccw
  arc A500 (96.0472, -63.5184) -> (97.2472, -63.5184) centre (96.6472, -63.5184) ccw
  arc A501 (97.2472, -63.5184) -> (96.0472, -63.5184) centre (96.6472, -63.5184) ccw
  arc A502 (194.7974, -80.3272) -> (195.9974, -80.3272) centre (195.3974, -80.3272) ccw
  arc A503 (195.9974, -80.3272) -> (194.7974, -80.3272) centre (195.3974, -80.3272) ccw
  arc A504 (191.2974, -82.5812) -> (192.4974, -82.5812) centre (191.8974, -82.5812) ccw
  arc A505 (192.4974, -82.5812) -> (191.2974, -82.5812) centre (191.8974, -82.5812) ccw
  arc A506 (194.7974, -23.1516) -> (195.9974, -23.1516) centre (195.3974, -23.1516) ccw
  arc A507 (195.9974, -23.1516) -> (194.7974, -23.1516) centre (195.3974, -23.1516) ccw
  arc A508 (192.4974, -25.4057) -> (191.2974, -25.4057) centre (191.8974, -25.4057) ccw
  arc A509 (191.2974, -25.4057) -> (192.4974, -25.4057) centre (191.8974, -25.4057) ccw
  arc A510 (81.6972, -80.3272) -> (80.4972, -80.3272) centre (81.0972, -80.3272) ccw
  arc A511 (80.4972, -80.3272) -> (81.6972, -80.3272) centre (81.0972, -80.3272) ccw
  arc A512 (78.1972, -82.5812) -> (76.9972, -82.5812) centre (77.5972, -82.5812) ccw
  arc A513 (76.9972, -82.5812) -> (78.1972, -82.5812) centre (77.5972, -82.5812) ccw
  arc A514 (81.6972, -42.2017) -> (80.4972, -42.2017) centre (81.0972, -42.2017) ccw
  arc A515 (80.4972, -42.2017) -> (81.6972, -42.2017) centre (81.0972, -42.2017) ccw
  arc A516 (78.1972, -44.4557) -> (76.9972, -44.4557) centre (77.5972, -44.4557) ccw
  arc A517 (76.9972, -44.4557) -> (78.1972, -44.4557) centre (77.5972, -44.4557) ccw
  arc A518 (81.6972, -23.1516) -> (80.4972, -23.1516) centre (81.0972, -23.1516) ccw
  arc A519 (80.4972, -23.1516) -> (81.6972, -23.1516) centre (81.0972, -23.1516) ccw
  arc A520 (76.9972, -25.4057) -> (78.1972, -25.4057) centre (77.5972, -25.4057) ccw
  arc A521 (78.1972, -25.4057) -> (76.9972, -25.4057) centre (77.5972, -25.4057) ccw
  arc A522 (81.6972, -61.2644) -> (80.4972, -61.2644) centre (81.0972, -61.2644) ccw
  arc A523 (80.4972, -61.2644) -> (81.6972, -61.2644) centre (81.0972, -61.2644) ccw
  arc A524 (78.1972, -63.5184) -> (76.9972, -63.5184) centre (77.5972, -63.5184) ccw
  arc A525 (76.9972, -63.5184) -> (78.1972, -63.5184) centre (77.5972, -63.5184) ccw
  arc A526 (61.4471, -80.3272) -> (62.6471, -80.3272) centre (62.0471, -80.3272) ccw
  arc A527 (62.6471, -80.3272) -> (61.4471, -80.3272) centre (62.0471, -80.3272) ccw
  arc A528 (57.9471, -82.5812) -> (59.1471, -82.5812) centre (58.5471, -82.5812) ccw
  arc A529 (59.1471, -82.5812) -> (57.9471, -82.5812) centre (58.5471, -82.5812) ccw
  arc A530 (61.4471, -61.2644) -> (62.6471, -61.2644) centre (62.0471, -61.2644) ccw
  arc A531 (62.6471, -61.2644) -> (61.4471, -61.2644) centre (62.0471, -61.2644) ccw
  arc A532 (59.1471, -63.5184) -> (57.9471, -63.5184) centre (58.5471, -63.5184) ccw
  arc A533 (57.9471, -63.5184) -> (59.1471, -63.5184) centre (58.5471, -63.5184) ccw
  arc A534 (62.6471, -42.2017) -> (61.4471, -42.2017) centre (62.0471, -42.2017) ccw
  arc A535 (61.4471, -42.2017) -> (62.6471, -42.2017) centre (62.0471, -42.2017) ccw
  arc A536 (57.9471, -44.4557) -> (59.1471, -44.4557) centre (58.5471, -44.4557) ccw
  arc A537 (59.1471, -44.4557) -> (57.9471, -44.4557) centre (58.5471, -44.4557) ccw
  arc A538 (43.5971, -61.2644) -> (42.3971, -61.2644) centre (42.9971, -61.2644) ccw
  arc A539 (42.3971, -61.2644) -> (43.5971, -61.2644) centre (42.9971, -61.2644) ccw
  arc A540 (40.0971, -63.5184) -> (38.8971, -63.5184) centre (39.4971, -63.5184) ccw
  arc A541 (38.8971, -63.5184) -> (40.0971, -63.5184) centre (39.4971, -63.5184) ccw
  arc A542 (42.3971, -80.3272) -> (43.5971, -80.3272) centre (42.9971, -80.3272) ccw
  arc A543 (43.5971, -80.3272) -> (42.3971, -80.3272) centre (42.9971, -80.3272) ccw
  arc A544 (38.8971, -82.5812) -> (40.0971, -82.5812) centre (39.4971, -82.5812) ccw
  arc A545 (40.0971, -82.5812) -> (38.8971, -82.5812) centre (39.4971, -82.5812) ccw
  arc A546 (24.547, -80.3272) -> (23.347, -80.3272) centre (23.947, -80.3272) ccw
  arc A547 (23.347, -80.3272) -> (24.547, -80.3272) centre (23.947, -80.3272) ccw
  arc A548 (21.047, -82.5812) -> (19.847, -82.5812) centre (20.447, -82.5812) ccw
  arc A549 (19.847, -82.5812) -> (21.047, -82.5812) centre (20.447, -82.5812) ccw
  arc A550 (4.297, -80.3272) -> (5.497, -80.3272) centre (4.897, -80.3272) ccw
  arc A551 (5.497, -80.3272) -> (4.297, -80.3272) centre (4.897, -80.3272) ccw
  arc A552 (0.797, -82.5812) -> (1.997, -82.5812) centre (1.397, -82.5812) ccw
  arc A553 (1.997, -82.5812) -> (0.797, -82.5812) centre (1.397, -82.5812) ccw
  arc A554 (62.6471, -23.1516) -> (61.4471, -23.1516) centre (62.0471, -23.1516) ccw
  arc A555 (61.4471, -23.1516) -> (62.6471, -23.1516) centre (62.0471, -23.1516) ccw
  arc A556 (59.1471, -25.4057) -> (57.9471, -25.4057) centre (58.5471, -25.4057) ccw
  arc A557 (57.9471, -25.4057) -> (59.1471, -25.4057) centre (58.5471, -25.4057) ccw
  arc A558 (42.3971, -42.2017) -> (43.5971, -42.2017) centre (42.9971, -42.2017) ccw
  arc A559 (43.5971, -42.2017) -> (42.3971, -42.2017) centre (42.9971, -42.2017) ccw
  arc A560 (40.0971, -44.4557) -> (38.8971, -44.4557) centre (39.4971, -44.4557) ccw
  arc A561 (38.8971, -44.4557) -> (40.0971, -44.4557) centre (39.4971, -44.4557) ccw
  arc A562 (43.5971, -23.1516) -> (42.3971, -23.1516) centre (42.9971, -23.1516) ccw
  arc A563 (42.3971, -23.1516) -> (43.5971, -23.1516) centre (42.9971, -23.1516) ccw
  arc A564 (38.8971, -25.4057) -> (40.0971, -25.4057) centre (39.4971, -25.4057) ccw
  arc A565 (40.0971, -25.4057) -> (38.8971, -25.4057) centre (39.4971, -25.4057) ccw
  arc A566 (23.347, -23.1516) -> (24.547, -23.1516) centre (23.947, -23.1516) ccw
  arc A567 (24.547, -23.1516) -> (23.347, -23.1516) centre (23.947, -23.1516) ccw
  arc A568 (19.847, -25.4057) -> (21.047, -25.4057) centre (20.447, -25.4057) ccw
  arc A569 (21.047, -25.4057) -> (19.847, -25.4057) centre (20.447, -25.4057) ccw
  arc A570 (24.547, -61.2644) -> (23.347, -61.2644) centre (23.947, -61.2644) ccw
  arc A571 (23.347, -61.2644) -> (24.547, -61.2644) centre (23.947, -61.2644) ccw
  arc A572 (21.047, -63.5184) -> (19.847, -63.5184) centre (20.447, -63.5184) ccw
  arc A573 (19.847, -63.5184) -> (21.047, -63.5184) centre (20.447, -63.5184) ccw
  arc A574 (23.347, -42.2017) -> (24.547, -42.2017) centre (23.947, -42.2017) ccw
  arc A575 (24.547, -42.2017) -> (23.347, -42.2017) centre (23.947, -42.2017) ccw
  arc A576 (19.847, -44.4557) -> (21.047, -44.4557) centre (20.447, -44.4557) ccw
  arc A577 (21.047, -44.4557) -> (19.847, -44.4557) centre (20.447, -44.4557) ccw
  arc A578 (5.497, -23.1516) -> (4.297, -23.1516) centre (4.897, -23.1516) ccw
  arc A579 (4.297, -23.1516) -> (5.497, -23.1516) centre (4.897, -23.1516) ccw
  arc A580 (1.997, -25.4057) -> (0.797, -25.4057) centre (1.397, -25.4057) ccw
  arc A581 (0.797, -25.4057) -> (1.997, -25.4057) centre (1.397, -25.4057) ccw
  arc A582 (4.297, -42.2017) -> (5.497, -42.2017) centre (4.897, -42.2017) ccw
  arc A583 (5.497, -42.2017) -> (4.297, -42.2017) centre (4.897, -42.2017) ccw
  arc A584 (1.997, -44.4557) -> (0.797, -44.4557) centre (1.397, -44.4557) ccw
  arc A585 (0.797, -44.4557) -> (1.997, -44.4557) centre (1.397, -44.4557) ccw
  arc A586 (4.297, -61.2644) -> (5.497, -61.2644) centre (4.897, -61.2644) ccw
  arc A587 (5.497, -61.2644) -> (4.297, -61.2644) centre (4.897, -61.2644) ccw
  arc A588 (1.997, -63.5184) -> (0.797, -63.5184) centre (1.397, -63.5184) ccw
  arc A589 (0.797, -63.5184) -> (1.997, -63.5184) centre (1.397, -63.5184) ccw
  arc A590 (213.8474, -61.2644) -> (215.0474, -61.2644) centre (214.4474, -61.2644) ccw
  arc A591 (215.0474, -61.2644) -> (213.8474, -61.2644) centre (214.4474, -61.2644) ccw
  arc A592 (211.5474, -63.5184) -> (210.3474, -63.5184) centre (210.9474, -63.5184) ccw
  arc A593 (210.3474, -63.5184) -> (211.5474, -63.5184) centre (210.9474, -63.5184) ccw